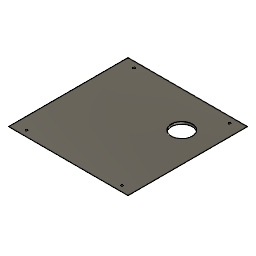
BBD - 200x200 mm (Autodesk Fusion 360 design; units mm, degrees)
part number: 2026-03-31-14-11-04-905
Autodesk Fusion 360 part; units mm, degrees
sketch "Esquisse1" plane through (0, 0, 0) normal (0, 0, 1) x (1, 0, 0)
  line L0 (0, 0) -> (200, 0)
  line L1 (200, 0) -> (200, 200)
  line L2 (200, 200) -> (0, 200)
  line L3 (0, 200) -> (0, 0)
  dimension "d18" = 200
  dimension "d19" = 200
  constraint horizontal L0
  constraint vertical L1
  constraint horizontal L2
  constraint vertical L3
  constraint coincident L0.start L3.end
  measures "d18" distance of L0 L2
  measures "d19" distance of L1 L3
extrude "Extrusion1" add sketch "Esquisse1" along normal blind 4
chamfer "Chanfrein1" distance 4 angle 45 1 faces at (66.6667, 133.3333, 0)
sketch "Esquisse2" plane through (0, 0, 4) normal (0, 0, 1) x (-1, 0, 0)
  circle A0 centre (-20, -190) radius 1.5
  circle A1 centre (-180, -190) radius 1.5
  circle A2 centre (-180, -10) radius 1.5
  circle A3 centre (-20, -10) radius 1.5
  line L0 (-3.4717, 2.3062) -> (-20, -10)
  line L1 (-200, 0) -> (-180, -10)
  line L2 (-200, 0) -> (-297.1716, 0) construction
  line L3 (-3.5105, -205.8754) -> (-20, -190)
  line L4 (-200, -200) -> (-180, -190)
  line L5 (-200, -200) -> (-297.1716, -200) construction
  line L6 (0, -200) -> (0, 0)
  line L7 (0, 0) -> (-200, 0)
  line L8 (-200, 0) -> (-200, -200)
  line L9 (-200, -200) -> (0, -200)
  line L10 (-20, -190) -> (-20, -200)
  line L11 (0, -190) -> (-20, -190)
  line L12 (-180, -190) -> (-200, -190)
  line L13 (-180, -190) -> (-180, -200)
  line L14 (-180, -10) -> (-200, -10)
  line L15 (-180, -10) -> (-180, 0)
  line L16 (-20, -10) -> (-20, 0)
  line L17 (-20, -10) -> (0, -10)
  dimension "d10" = 3
  dimension "d11" = 3
  dimension "d12" = 3
  dimension "d13" = 3
  dimension "d33" = 20
  dimension "d34" = 10
  dimension "d35" = 10
  dimension "d36" = 20
  dimension "d37" = 10
  dimension "d38" = 20
  dimension "d39" = 10
  dimension "d40" = 20
  constraint coincident A3.centre L0.end
  constraint horizontal L2
  constraint coincident A2.centre L1.end
  constraint coincident A0.centre L3.end
  constraint horizontal L5
  constraint coincident A1.centre L4.end
  constraint coincident L1.start L2.start
  constraint coincident L4.start L5.start
  constraint coincident L9 L10.end
  constraint perpendicular L9 L10
  constraint coincident L6 L11.start
  constraint perpendicular L10 L11
  constraint coincident L8 L12.end
  constraint perpendicular L8 L12
  constraint coincident L9 L13.end
  constraint perpendicular L9 L13
  constraint coincident L8 L14.end
  constraint perpendicular L8 L14
  constraint coincident L7 L15.end
  constraint perpendicular L7 L15
  constraint coincident L7 L16.end
  constraint perpendicular L7 L16
  constraint coincident L6 L17.end
  constraint perpendicular L6 L17
  measures "d10" diameter of A0
  measures "d11" diameter of A1
  measures "d12" diameter of A2
  measures "d13" diameter of A3
  measures "d33" distance of A3.centre L17.end
  measures "d34" distance of A3.centre L16.end
  measures "d35" distance of A2.centre L15.end
  measures "d36" distance of A2.centre L14.end
  measures "d37" distance of A1.centre L13.end
  measures "d38" distance of A1.centre L12.end
  measures "d39" distance of A0.centre L10.end
  measures "d40" distance of A0.centre L11.start
extrude "Extrusion2" cut sketch "Esquisse2" against normal blind 14 contours A0 L10 L11 | A0 L3 L11 | A0 L3 L10 | A3 L0 L17 | A3 L16 L17 | A1 L12 L13 | A1 L4 L13 | A3 L0 L16 | A1 L4 L12 | A2 L14 L15 | A2 L1 L14 | A2 L1 L15
thread "Filetage1" "ISO Metric profile 4.0 M4x0.7 M4x0.7 6H" major diameter 4.1095 minor diameter 3.332 pitch 0.7 angle 60 resizes the face on face at (21.4536, 189.6299, 2.6667)
thread "Filetage2" "ISO Metric profile 4.0 M4x0.7 M4x0.7 6H" major diameter 4.1095 minor diameter 3.332 pitch 0.7 angle 60 resizes the face on face at (18.5075, 10.1494, 1.3333)
thread "Filetage3" "ISO Metric profile 4.0 M4x0.7 M4x0.7 6H" major diameter 4.1095 minor diameter 3.332 pitch 0.7 angle 60 resizes the face on face at (180.6169, 8.6327, 1.3333)
thread "Filetage4" "ISO Metric profile 4.0 M4x0.7 M4x0.7 6H" major diameter 4.1095 minor diameter 3.332 pitch 0.7 angle 60 resizes the face on face at (179.1244, 188.7821, 1.3333)
sketch "Esquisse3" plane through (0, 0, 4) normal (0, 0, 1) x (-1, 0, 0)
  circle A0 centre (-180, -190) radius 1.666
  circle A1 centre (-180, -10) radius 1.666
  circle A2 centre (-20, -190) radius 1.666
  circle A3 centre (-20, -10) radius 1.666
  line L0 (0, -200) -> (0, 0)
  line L1 (0, 0) -> (-200, 0)
  line L2 (-200, 0) -> (-200, -200)
  line L3 (-200, -200) -> (0, -200)
  circle A4 centre (-150, -140) radius 17.5
  point P0 (-150, -140)
  dimension "d28" = 60
  dimension "d29" = 50
  dimension "d30" = 35
  constraint coincident P0 A4.centre
  measures "d28" distance of L3 P0
  measures "d29" distance of L2 P0
  measures "d30" diameter of A4
extrude "Extrusion3" cut sketch "Esquisse3" against normal blind 10 contours A4
move_face "DécalerLesFaces1" offset -0.05 1 faces at (18.3423, 10.1659, 1.3333)
move_face "DécalerLesFaces2" offset -0.05 1 faces at (18.3423, 190.1659, 1.3333)
move_face "DécalerLesFaces3" offset -0.05 1 faces at (178.3423, 190.1659, 1.3333)
move_face "DécalerLesFaces4" offset -0.05 1 faces at (178.672, 8.9941, 2.6667)
